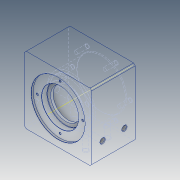
# Autodesk Inventor part: 200-10-ROCKER-BEARING-01
Saved by Autodesk Inventor 2018.1 (Build 221171000, 171)
## iProperties
Manager: Martin Fees
Company: NRBDL
Created: 2017-10-25
Part Number: 200-10-ROCKER-BEARING-01
Material: Aluminium 6061
Document SubType Name: Modeling
Designer: Martin Fees
Density: 2.7 g/cm^3
Appearance: Aluminium - flach
Project: Mobiler Rettungsroboter
Description: Rocker Achsaufnahme inklusive Lagerung
Engineer: Martin Fees
Authority: Martin Fees
Stock Number: 200-10-ROCKER-BEARING-01
Mass: 1000.27 g
Surface Area: 570.153 cm^2
Volume: 370.471 cm^3
Author: Martin Fees
Title: Rocker Achsaufnahme inklusive Lagerung
Subject: Roboter
Revision Number: 1
Autodesk Inventor part; units mm, degrees
ref_plane "YZ Plane" through (0, 0, 0) normal (1, 0, 0) x (0, 1, 0)
ref_plane "XZ Plane" through (0, 0, 0) normal (0, 1, 0) x (-1, 0, 0)
ref_plane "XY Plane" through (0, 0, 0) normal (0, 0, 1) x (1, 0, 0)
sketch "Skizze1" plane through (0, 0, 0) normal (0, 1, 0) x (-1, 0, 0)
  line L0 (0, -50) -> (-50, -50)
  line L1 (-50, -50) -> (-50, 50)
  line L2 (-50, 50) -> (0, 50)
  line L3 (0, -50) -> (50, -50)
  line L4 (50, -50) -> (50, 50)
  line L5 (50, 50) -> (0, 50)
  line L6 (-122.5, 0) -> (122.5, 0) construction
  line L7 (0, -77.2) -> (0, 113.2) construction
  dimension "d1" = 100
  dimension "d3" = 100
  constraints: 12 end point, 3 horizontal, 1 parallel, 1 point on line, 1 vertical, 2 other
  measures "d1" distance between parallel lines of L0 L2
  measures "d3" distance between parallel lines of L1 L4
extrude "Grundkoerper" add sketch "Skizze1" along normal mid plane 65
sketch "Skizze2" plane through (0, -32.5, 0) normal (0, -1, 0) x (1, 0, 0)
  line L0 (-50, -50) -> (50, -50) projected
  line L1 (50, 50) -> (-50, 50) projected
  point P0 (0, 0)
  point P1 (0, 0)
  point P2 (-87.5, 0)
  point P3 (87.5, 0)
  dimension "d8" = 0
  constraints: 1 other
  measures "d8" distance of point (0, 0) point (0, 0)
sketch "Skizze3" plane through (0, 0, 0) normal (1, 0, 0) x (0, 1, 0)
  line L0 (49, 0) -> (-49, 0) construction
  line L1 (-32.5, 50) -> (-32.5, -50) construction
  line L2 (32.5, -50) -> (32.5, 50) construction
  line L3 (32.5, 36) -> (-12.5, 36)
  line L4 (-12.5, 36) -> (-12.5, 32.25)
  line L5 (-17.5, 18) -> (-32.5, 18)
  line L6 (-32.5, -50) -> (-32.5, 50) projected
  line L7 (-32.5, 18) -> (-32.5, 0)
  line L8 (-32.5, 0) -> (32.5, 0)
  line L9 (32.5, 0) -> (32.5, 36)
  line L10 (-12.5, 32.25) -> (-17.5, 32.25)
  line L11 (-17.5, 32.25) -> (-17.5, 18)
  point P0 (0, 0)
  dimension "d9" = 45
  dimension "d10" = 72
  dimension "d11" = 36
  dimension "d33" = 5
  dimension "d34" = 64.5
  constraints: 16 end point, 4 perpendicular, 4 point on line, 2 horizontal, 2 midpoint
  measures "d9" distance between parallel lines of L2 L4
  measures "d10" diameter of L3 L0
  measures "d11" diameter of L5 L0
  measures "d33" distance of L4.end L10.end
  measures "d34" diameter of L10 L0
revolve "Lagersitz" cut sketch "Skizze3" angle 360 about axis through (0, -32.5, 0) along (0, -1, 0)
sketch "Skizze_Lagersitz" plane through (0, 0, 0) normal (1, 0, 0) x (0, 1, 0)
  line L0 (-12.5, 36) -> (32.5, 36) projected
  line L1 (-12.5, -36) -> (-12.5, 36) projected
  line L2 (-17.5, 32.25) -> (-12.5, 32.25) projected
  line L3 (-17.5, -32.25) -> (-17.5, 32.25) projected
  line L4 (-32.5, 18) -> (-17.5, 18) projected
  line L5 (-32.5, -18) -> (-17.5, -18) projected
  line L6 (-17.5, -32.25) -> (-12.5, -32.25) projected
  line L7 (-12.5, -36) -> (32.5, -36) projected
  line L8 (32.5, 36) -> (32.5, -36) projected
  line L9 (32.5, 50) -> (32.5, -50) projected
  line L10 (30, -50) -> (30, 0) projected
  line L11 (-32.5, -18) -> (-32.5, 18) projected
  line L12 (-32.5, 50) -> (-32.5, -50) projected
  line L13 (-32.5, -50) -> (-32.5, 50) projected
  line L14 (-12.5, -36) -> (-12.5, 36) projected
  point P0 (0, 0)
  point P1 (30, 86)
  point P2 (30, 14)
  point P3 (-30, 32)
  point P4 (-30, 68)
  constraints: 2 other
sketch "Skizze10" plane through (0, 0, 0) normal (1, 0, 0) x (0, 1, 0)
  line L0 (49, 0) -> (-49, 0) projected
  line L1 (-32.5, 18) -> (-17.5, 18) construction
  line L2 (-32.5, -50) -> (-32.5, 50) construction
  line L3 (-17.5, -32.25) -> (-17.5, 32.25) construction
  line L4 (-32.5, 50) -> (-32.5, -50) projected
  line L5 (-29.5, 27.5) -> (-21.7, 27.5)
  line L6 (-21.2, 27) -> (-21.2, 22.5)
  line L7 (-21.2, 22.5) -> (-17.5, 22.5)
  line L8 (-17.5, 22.5) -> (-17.5, 18)
  line L9 (-32.5, 40) -> (-32.5, 0)
  line L10 (-32.5, 0) -> (-17.5, 0)
  line L11 (-17.5, 0) -> (-17.5, 22.5)
  arc A0 (-21.2, 27) -> (-21.7, 27.5) centre (-21.7, 27) ccw
  line L12 (-29.5, 27.5) -> (-29.5, 40)
  line L13 (-29.5, 40) -> (-32.5, 40)
  point P0 (0, 0)
  dimension "d117" = 55
  dimension "d118" = 0.5
  dimension "d119" = 45
  dimension "d124" = 8.3
  dimension "d125" = 3
  dimension "d126" = 80
  constraints: 18 end point, 3 perpendicular, 2 collinear, 2 midpoint, 2 point on circle, 2 point on line, 2 tangent, 1 centre point, 1 horizontal, 1 vertical
  measures "d117" diameter of L5 L0
  measures "d118" radius of A0
  measures "d119" diameter of L7 L0
  measures "d124" distance between parallel lines of L12 L6
  measures "d125" distance of L9.start L12.end
  measures "d126" diameter of L13 L0
revolve "RWDR" cut sketch "Skizze10" angle 360 about axis through (0, -32.5, 0) along (0, -1, 0)
sketch "Skizze_RWDR" plane through (0, 0, 0) normal (1, 0, 0) x (0, 1, 0)
  line L0 (-32.5, -40) -> (-32.5, 40) projected
  line L1 (-32.5, 40) -> (-29.5, 40) projected
  line L2 (-29.5, -40) -> (-29.5, 40) projected
  line L3 (-32.5, -40) -> (-29.5, -40) projected
  line L4 (-29.5, 27.5) -> (-21.7, 27.5) projected
  line L5 (-21.2, -27) -> (-21.2, 27) projected
  line L6 (-29.5, -27.5) -> (-21.7, -27.5) projected
  arc A0 (-21.7, -27.5) -> (-21.2, -27) centre (-21.7, -27) ccw projected
  arc A1 (-21.2, 27) -> (-21.7, 27.5) centre (-21.7, 27) ccw projected
  line L7 (-21.2, 22.5) -> (-17.5, 22.5) projected
  line L8 (-21.2, -22.5) -> (-17.5, -22.5) projected
  line L9 (-17.5, 22.5) -> (-17.5, -22.5) projected
  point P0 (0, 0)
sketch "Skizze5" plane through (0, 32.5, 0) normal (0, 1, 0) x (1, 0, 0)
  circle A0 centre (0, 0) radius 36 construction
  circle A1 centre (0, 0) radius 43 construction
  line L0 (-50, -50) -> (50, -50) construction
  line L1 (50, 50) -> (-50, 50) projected
  line L2 (-50, 50) -> (50, 50) construction
  line L3 (0, 77.2) -> (0, -113.2) construction
  line L4 (0, 0) -> (21.5, -37.2391) construction
  point P0 (43, 0)
  point P1 (21.5, 37.2391)
  point P2 (-21.5, 37.2391)
  point P3 (-43, 0)
  point P4 (-21.5, -37.2391)
  dimension "d40" = 86
  dimension "d38" = 100
  dimension "d39" = 72
  dimension "d110" = 30
  dimension "d114" = 360
  constraints: 2 end point, 1 coincident, 10 other
  measures "d38" distance between parallel lines of L1 L0
  measures "d39" diameter of A0
  measures "d110" angle of L3 L4
hole "M6_Boh_Lagerpresse" at (21.5, 32.5, 37.2391) at (43, 32.5, 0) at (21.5, 32.5, -37.2391) at (-21.5, 32.5, -37.2391) at (-43, 32.5, 0) at (-21.5, 32.5, 37.2391) direction (0, -1, 0) diameter 4.917 depth 17.1 tip angle 118 countersink diameter 6 countersink angle 90 thread size "M6x1" class "6H" standard "ISO Metric profile"
sketch "Skizze11" plane through (0, -29.5, 0) normal (0, -1, 0) x (1, 0, 0)
  circle A0 centre (0, 0) radius 40 construction
  circle A1 centre (0, 0) radius 27.5 construction
  circle A2 centre (0, 0) radius 33.75 construction
  line L0 (0, 113.2) -> (0, -77.2) construction
  line L1 (-122.5, 0) -> (122.5, 0) projected
  point P0 (0, 33.75)
  point P1 (-33.75, 0)
  point P2 (0, -33.75)
  point P3 (33.75, 0)
  dimension "d129" = 67.5
  dimension "d127" = 55
  dimension "d128" = 80
  dimension "d132" = 360
  constraints: 1 coincident, 1 point on line, 1 vertical alignment, 7 other
  measures "d127" diameter of A1
  measures "d128" diameter of A0
hole "M3_RWDR_Fixierung" at (0, -29.5, 33.75) at (-33.75, -29.5, 0) at (0, -29.5, -33.75) at (33.75, -29.5, 0) direction (0, 1, 0) diameter 2.459 depth 8.8 tip angle 118 countersink diameter 3 countersink angle 90 thread size "M3x0.5" class "6H" standard "ISO Metric profile"
sketch "Skizze8" plane through (50, 32.5, -50) normal (0, 0, -1) x (-1, 0, 0)
  line L0 (0, 0) -> (100, 0) construction
  line L1 (100, -65) -> (0, -65) construction
  line L2 (0, 0) -> (0, -65) construction
  line L3 (100, 0) -> (100, -65) construction
  line L4 (50, -84.5) -> (50, 17) construction
  line L5 (-72.5, -32.5) -> (172.5, -32.5) construction
  point P0 (50, -32.5)
  point P1 (25, -16.25)
  point P2 (75, -16.25)
  point P3 (25, -48.75)
  point P4 (75, -48.75)
  dimension "d81" = 100
  dimension "d82" = 50
  dimension "d83" = 65
  dimension "d84" = 32.5
  constraints: 2 symmetric about line, 1 horizontal alignment
  measures "d81" distance of L1.start L1.end
  measures "d82" distance of point (75, -16.25) point (25, -16.25)
  measures "d83" distance between parallel lines of L0 L1
  measures "d84" distance of point (25, -48.75) point (25, -16.25)
hole "M8_Boh_Fixierung_1" at (25, 16.25, -50) at (-25, 16.25, -50) at (25, -16.25, -50) at (-25, -16.25, -50) direction (0, 0, 1) diameter 6.647 depth 18.2 tip angle 118 countersink diameter 8 countersink angle 90 thread size "M8x1.25" class "6H" standard "ISO Metric profile"
sketch "Skizze9" plane through (50, -32.5, -50) normal (1, 0, 0) x (0, 0, -1)
  line L0 (-50, 81.5) -> (-50, -16.5) construction
  line L1 (0, 65) -> (0, 0) construction
  line L2 (-100, 65) -> (0, 65) construction
  line L3 (0, 0) -> (-100, 0) construction
  line L4 (-163.2, 32.5) -> (27.2, 32.5) construction
  point P0 (-50, 32.5)
  point P1 (-25, 16.25)
  point P2 (-25, 48.75)
  dimension "d92" = 32.5
  dimension "d93" = 65
  dimension "d94" = 50
  dimension "d95" = 25
  constraints: 1 symmetric about line, 1 other
  measures "d92" distance of point (-25, 48.75) point (-25, 16.25)
  measures "d93" distance of L2.end L3.start
  measures "d94" distance of the line from the sketch origin of L0
hole "M8_Boh_Fixierung_2" at (50, -16.25, -25) at (50, 16.25, -25) direction (-1, 0, 0) diameter 6.647 depth 18.2 tip angle 118 countersink diameter 8 countersink angle 90 thread size "M8x1.25" class "6H" standard "ISO Metric profile"
mirror "M8_Boh_Fixierung_2_Spiegel" about plane through (0, 0, 0) normal (1, 0, 0) of "M8_Boh_Fixierung_2"
chamfer "Fase_Lagersitz" distance 0.25 angle 45 1 edges at (0, -12.5, -32.25)
chamfer "Fase_Deckel" distance 1 angle 45 1 edges at (0, 32.5, -36)
chamfer "Fase_Allgemein" distance 2.5 angle 45 4 edges at (50, 0, 50) (-50, 0, 50) (50, 0, -50) (-50, 0, -50)
chamfer "Fase_RWDR" distance 0.2 angle 45 2 edges at (0, -29.5, -27.5) (0, -32.5, -40)
equation "\"d40\" = 0.5 * d38 + 0.5 * d39"
equation "\"d129\" = 0.5 * d128 + 0.5 * d127"
equation "\"d82\" = 0.5 * d81"
equation "\"d84\" = 0.5 * d83"
equation "\"d92\" = 0.5 * d93"
equation "\"d95\" = 0.5 * d94"
